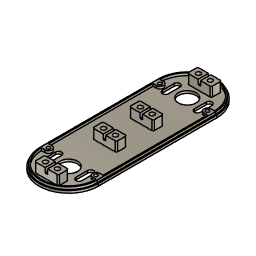
TRARM02_Link2A_100x50x2 (Autodesk Fusion 360 design; units mm, degrees)
Autodesk Fusion 360 part; units mm, degrees
sketch "스케치1" plane through (0, 0, 0) normal (0, 0, 1) x (1, 0, 0)
  line L0 (25, 100) -> (25, 0)
  line L1 (-25, 100) -> (-25, 0)
  arc A0 (25, 100) -> (-25, 100) centre (0, 100) ccw
  arc A1 (-25, 0) -> (25, 0) centre (0, 0) ccw
  dimension "d1" = 50
  dimension "d140" = 100
  constraint coincident A1.centre origin
  constraint vertical A1.centre A0.centre
  constraint vertical L0
  constraint tangent L1 A0
  constraint parallel L0 L1
  constraint horizontal A1.centre L1.end
  constraint horizontal A1.centre L0.end
  measures "d1" diameter of A1
  measures "d140" distance of L1.start L1.end
extrude "돌출1" add sketch "스케치1" along normal blind 2
sketch "스케치2" plane through (0, 0, 2) normal (0, 0, 1) x (-1, 0, 0)
  circle A0 centre (0, 0) radius 7.5
  circle A1 centre (0, -100) radius 7.5
  point P0 (25, -100)
  dimension "d150" = 100
  dimension "d151" = 15
  constraint coincident A0.centre origin
  constraint equal A0 A1
  constraint vertical A0.centre A1.centre
  measures "d150" distance of A0.centre A1.centre
  measures "d151" diameter of A0
extrude "돌출18" cut sketch "스케치2" against normal blind 2
sketch "스케치17" plane through (0, 0, 2) normal (0, 0, 1) x (-1, 0, 0)
  line L0 (10, -118.8) -> (-10, -118.8)
  line L1 (-10, -118.8) -> (-10, -110.2)
  line L2 (-10, -110.2) -> (10, -110.2)
  line L3 (10, -110.2) -> (10, -118.8)
  line L4 (10, -69.8) -> (-10, -69.8)
  line L5 (-10, -69.8) -> (-10, -61.2)
  line L6 (-10, -61.2) -> (10, -61.2)
  line L7 (10, -61.2) -> (10, -69.8)
  line L8 (10, -38.8) -> (-10, -38.8)
  line L9 (-10, -38.8) -> (-10, -30.2)
  line L10 (-10, -30.2) -> (10, -30.2)
  line L11 (10, -30.2) -> (10, -38.8)
  line L12 (10, 10.2) -> (-10, 10.2)
  line L13 (-10, 10.2) -> (-10, 18.8)
  line L14 (-10, 18.8) -> (10, 18.8)
  line L15 (10, 18.8) -> (10, 10.2)
  circle A0 centre (0, -100) radius 7.5
  circle A1 centre (-5, 14.5) radius 2.1 construction
  circle A2 centre (5, 14.5) radius 2.1 construction
  dimension "d154" = 20
  dimension "d160" = 10
  dimension "d161" = 10.2
  dimension "d162" = 10.2
  dimension "d163" = 30.2
  dimension "d164" = 30.2
  dimension "d165" = 4.2
  dimension "d166" = 14.5
  dimension "d167" = 10
  dimension "d168" = 5
  dimension "d169" = 4.3
  constraint horizontal L0
  constraint vertical L1
  constraint horizontal L2
  constraint vertical L3
  constraint horizontal L4
  constraint vertical L5
  constraint horizontal L6
  constraint vertical L7
  constraint horizontal L8
  constraint vertical L9
  constraint horizontal L10
  constraint vertical L11
  constraint horizontal L12
  constraint vertical L13
  constraint horizontal L14
  constraint vertical L15
  constraint equal L10 L14
  constraint equal L6 L10
  constraint equal L2 L6
  constraint equal L1 L5
  constraint equal L5 L9
  constraint vertical L6.end L10.end
  constraint vertical L10.end L14.end
  constraint vertical L2.end L6.end
  constraint equal L9 L13
  constraint equal A1 A2
  constraint horizontal A1.centre A2.centre
  measures "d154" distance of L13.end L14.end
  measures "d160" horizontal distance of origin L13.end
  measures "d161" vertical distance of origin L12.start
  measures "d162" vertical distance of L2.end A0.centre
  measures "d163" vertical distance of L4.start A0.centre
  measures "d164" vertical distance of origin L10.end
  measures "d165" diameter of A1
  measures "d166" vertical distance of origin A1.centre
  measures "d167" distance of A1.centre A2.centre
  measures "d168" horizontal distance of origin A1.centre
  measures "d169" vertical distance of L13.end A1.centre
extrude "돌출19" add sketch "스케치17" along normal blind 8 contours L0 L1 L2 L3 | L4 L5 L6 L7 | L8 L9 L10 L11 | L12 L13 L14 L15
sketch "스케치18" plane through (0, 0, 10) normal (0, 0, 1) x (-1, 0, 0)
  circle A0 centre (5, 14.5) radius 1.95
  circle A1 centre (-5, 14.5) radius 1.95
  circle A2 centre (-5, -34.5) radius 1.95
  circle A3 centre (5, -34.5) radius 1.95
  circle A4 centre (-5, -65.5) radius 1.95
  circle A5 centre (5, -65.5) radius 1.95
  circle A6 centre (5, -114.5) radius 1.95
  circle A7 centre (-5, -114.5) radius 1.95
  circle A8 centre (0, -100) radius 7.5
  line L0 (1, 10.2) -> (-1, 10.2)
  line L1 (-1, 10.2) -> (-1, 18.8)
  line L2 (-1, 18.8) -> (1, 18.8)
  line L3 (1, 18.8) -> (1, 10.2)
  line L4 (10, 10.2) -> (-10, 10.2)
  line L5 (-10, 18.8) -> (10, 18.8)
  line L6 (1, -30.2) -> (-1, -30.2)
  line L7 (-1, -30.2) -> (-1, -38.8)
  line L8 (-1, -38.8) -> (1, -38.8)
  line L9 (1, -38.8) -> (1, -30.2)
  line L10 (-10, -30.2) -> (10, -30.2)
  line L11 (10, -38.8) -> (-10, -38.8)
  line L12 (1, -69.8) -> (-1, -69.8)
  line L13 (-1, -69.8) -> (-1, -61.2)
  line L14 (-1, -61.2) -> (1, -61.2)
  line L15 (1, -61.2) -> (1, -69.8)
  line L16 (10, -69.8) -> (-10, -69.8)
  line L17 (-10, -61.2) -> (10, -61.2)
  line L18 (1, -118.8) -> (-1, -118.8)
  line L19 (-1, -118.8) -> (-1, -110.2)
  line L20 (-1, -110.2) -> (1, -110.2)
  line L21 (1, -110.2) -> (1, -118.8)
  line L22 (10, -118.8) -> (-10, -118.8)
  line L23 (-10, -110.2) -> (10, -110.2)
  dimension "d172" = 14.5
  dimension "d173" = 3.9
  dimension "d174" = 10
  dimension "d175" = 5
  dimension "d177" = 49
  dimension "d178" = 49
  dimension "d179" = 14.5
  dimension "d182" = 2
  dimension "d183" = 1
  constraint horizontal A0.centre A1.centre
  constraint equal A0 A1
  constraint vertical A4.centre A7.centre
  constraint vertical A2.centre A4.centre
  constraint vertical A1.centre A2.centre
  constraint equal A1 A4
  constraint equal A2 A4
  constraint equal A4 A7
  constraint equal A5 A6
  constraint equal A2 A3
  constraint vertical A5.centre A6.centre
  constraint vertical A3.centre A5.centre
  constraint vertical A0.centre A3.centre
  constraint horizontal A2.centre A3.centre
  constraint horizontal A4.centre A5.centre
  constraint horizontal A6.centre A7.centre
  constraint equal A6 A7
  constraint horizontal L0
  constraint vertical L1
  constraint horizontal L2
  constraint vertical L3
  constraint coincident L1.end L5
  constraint coincident L0.start L4
  constraint horizontal L6
  constraint vertical L7
  constraint horizontal L8
  constraint vertical L9
  constraint coincident L7.end L11
  constraint coincident L6.start L10
  constraint vertical L0.end L6.end
  constraint vertical L0.start L6.start
  constraint horizontal L12
  constraint vertical L13
  constraint horizontal L14
  constraint vertical L15
  constraint coincident L13.end L17
  constraint coincident L12.start L16
  constraint vertical L7.end L13.end
  constraint vertical L8.end L14.end
  constraint horizontal L18
  constraint vertical L19
  constraint horizontal L20
  constraint vertical L21
  constraint coincident L19.end L23
  constraint coincident L18.start L22
  constraint vertical L12.end L19.end
  constraint vertical L12.start L20.end
  measures "d172" vertical distance of origin A1.centre
  measures "d173" diameter of A1
  measures "d174" distance of A0.centre A1.centre
  measures "d175" horizontal distance of origin A1.centre
  measures "d177" distance of A0.centre A3.centre
  measures "d178" distance of A5.centre A6.centre
  measures "d179" vertical distance of A7.centre A8.centre
  measures "d182" distance of L1.end L2.end
  measures "d183" horizontal distance of origin L1.end
extrude "돌출20" cut sketch "스케치18" against normal blind 5 contours A0 | A1 | A2 | A3 | A4 | A5 | A6 | A7
extrude "돌출21" cut sketch "스케치18" against normal blind 4 contours L0 L1 L2 L3 L4 L5 | L6 L7 L8 L9 L10 L11 | L12 L13 L14 L15 L16 L17 | L18 L19 L20 L21 L22 L23
sketch "스케치19" plane through (0, 0, 2) normal (0, 0, 1) x (-1, 0, 0)
  line L0 (25, -100) -> (25, 0) construction
  arc A0 (-25, -100) -> (25, -100) centre (0, -100) ccw construction
  line L1 (-25, 0) -> (-25, -100) construction
  arc A1 (25, 0) -> (-25, 0) centre (0, 0) ccw construction
  line L2 (24, -100) -> (24, 0)
  arc A2 (24, 0) -> (-24, 0) centre (0, 0) ccw
  line L3 (-24, 0) -> (-24, -100)
  arc A3 (-24, -100) -> (24, -100) centre (0, -100) ccw
  arc A4 (23, 0) -> (-23, 0) centre (0, 0) ccw
  line L4 (-23, -6) -> (-23, -94)
  arc A5 (-23, -100) -> (23, -100) centre (0, -100) ccw
  line L5 (-20, -6) -> (-23, -6)
  line L6 (-20, 0) -> (-23, 0)
  arc A6 (-20, -6) -> (-20, 0) centre (-20, -3) ccw
  line L7 (20, -6) -> (23, -6)
  line L8 (20, 0) -> (23, 0)
  line L9 (23, -94) -> (23, -6)
  arc A7 (20, 0) -> (20, -6) centre (20, -3) ccw
  line L10 (-20, -100) -> (-23, -100)
  line L11 (-20, -94) -> (-23, -94)
  arc A8 (-20, -100) -> (-20.0042, -94) centre (-20, -97) ccw
  line L12 (20, -100) -> (23, -100)
  line L13 (20, -94) -> (23, -94)
  arc A9 (20.0029, -94) -> (20, -100) centre (20, -97) ccw
  dimension "d186" = -1
  dimension "d192" = 6
  dimension "d193" = 3
  dimension "d195" = 20
  dimension "d196" = 20
  dimension "d198" = 3
  constraint equal A8 A9
  constraint equal A7 A9
  constraint equal A6 A7
  constraint horizontal A7.centre A6.centre
  constraint horizontal A9.centre A8.centre
  constraint vertical A7.centre A9.centre
  constraint vertical A6.centre A8.centre
  constraint perpendicular L4 L5
  constraint perpendicular L4 L6
  constraint concentric A1 A4
  constraint concentric A0 A5
  constraint tangent A4 L9
  constraint tangent A4 L4
  constraint tangent L4 A5
  constraint tangent A5 L9
  constraint perpendicular L7 L9
  constraint perpendicular L8 L9
  constraint equal L7 L8
  constraint equal L6 L7
  constraint equal L5 L6
  constraint coincident L11.start A8
  constraint perpendicular L4 L11
  constraint coincident L11 A8.end
  constraint coincident L13.start A9
  constraint perpendicular L9 L13
  constraint coincident L13 A9.start
  constraint equal L10 L11
  constraint equal L5 L10
  constraint horizontal A5.start A0.centre
  constraint horizontal A0.centre A5.end
  constraint horizontal L10
  constraint horizontal L12
  constraint equal L12 L13
  measures "d192" diameter of A6
  measures "d193" vertical distance of A1.centre A6.centre
  measures "d195" horizontal distance of A1.centre A6.centre
  measures "d196" horizontal distance of A1.centre A7.centre
  measures "d198" distance of L5.start L4.start
extrude "돌출22" add sketch "스케치19" along normal blind 2
sketch "스케치21" plane through (0, 0, 4) normal (0, 0, 1) x (-1, 0, 0)
  circle A0 centre (-20, -3) radius 1.5
  circle A1 centre (20, -3) radius 1.5
  circle A2 centre (-20, -97) radius 1.5
  arc A3 (-20, -100) -> (-20.0042, -94) centre (-20, -97) ccw
  circle A4 centre (20, -97) radius 1.5
  arc A5 (20.0029, -94) -> (20, -100) centre (20, -97) ccw
  arc A6 (-20, -6) -> (-20, 0) centre (-20, -3) ccw
  arc A7 (20, 0) -> (20, -6) centre (20, -3) ccw
  dimension "d199" = 3
  constraint concentric A2 A3
  constraint concentric A4 A5
  constraint equal A2 A4
  constraint equal A0 A2
  constraint equal A0 A1
  constraint concentric A0 A6
  constraint concentric A1 A7
  measures "d199" diameter of A0
extrude "돌출24" cut sketch "스케치21" against normal blind 4
chamfer "챔퍼5" distance 2 angle 45 4 edges at (21.3985, 3.5424, 0) (-18.6015, 3.5424, 0) (-18.6015, 97.5424, 0) (21.3985, 97.5424, 0)
fillet "필렛4" radius 1 16 edges at (10, -18.8, 6) (10, -10.2, 6) (10, 30.2, 6) (10, 38.8, 6) (10, 61.2, 6) (10, 69.8, 6) (10, 110.2, 6) (10, 118.8, 6) (-10, 118.8, 6) (-10, 110.2, 6) (-10, 69.8, 6) (-10, 61.2, 6) (-10, 38.8, 6) (-10, 30.2, 6) (-10, -10.2, 6) (-10, -18.8, 6)
sketch "스케치23" plane through (0, 0, 2) normal (0, 0, 1) x (-1, 0, 0)
  line L0 (-16, -5) -> (-16, 5)
  line L1 (-11, -5) -> (-11, 5)
  arc A0 (-16, -5) -> (-11, -5) centre (-13.5, -5) ccw
  arc A1 (-11, 5) -> (-16, 5) centre (-13.5, 5) ccw
  arc A2 (16, 5) -> (11, 5) centre (13.5, 5) ccw
  line L2 (11, -5) -> (11, 5)
  line L3 (16, -5) -> (16, 5)
  arc A3 (11, -5) -> (16, -5) centre (13.5, -5) ccw
  arc A4 (-11, -95) -> (-16, -95) centre (-13.5, -95) ccw
  line L4 (-16, -105) -> (-16, -95)
  arc A5 (-16, -105) -> (-11, -105) centre (-13.5, -105) ccw
  line L5 (-11, -105) -> (-11, -95)
  arc A6 (16, -95) -> (11, -95) centre (13.5, -95) ccw
  line L6 (11, -105) -> (11, -95)
  line L7 (16, -105) -> (16, -95)
  arc A7 (11, -105) -> (16, -105) centre (13.5, -105) ccw
  dimension "d212" = 10
  dimension "d213" = 2.5
  dimension "d214" = 5
  dimension "d215" = 13.5
  dimension "d216" = 10
  dimension "d218" = 13.5
  dimension "d221" = 10
  dimension "d222" = 2.5
  dimension "d223" = 10
  dimension "d224" = 95
  constraint equal A0 A1
  constraint tangent L0 A0
  constraint tangent L1 A1
  constraint tangent L0 A1
  constraint tangent L1 A0
  constraint vertical A0.centre A1.centre
  constraint equal A2 A3
  constraint tangent L2 A3
  constraint tangent A2 L3
  constraint tangent A2 L2
  constraint tangent L3 A3
  constraint vertical A3.centre A2.centre
  constraint horizontal A1.centre A2.centre
  constraint equal A0 A3
  constraint equal A4 A5
  constraint tangent L4 A5
  constraint tangent A4 L5
  constraint tangent A4 L4
  constraint tangent A5 L5
  constraint vertical A5.centre A4.centre
  constraint equal A6 A7
  constraint tangent L6 A7
  constraint tangent A6 L7
  constraint tangent A6 L6
  constraint tangent L7 A7
  constraint vertical A7.centre A6.centre
  constraint horizontal A4.centre A6.centre
  constraint equal A5 A7
  constraint vertical A0.centre A4.centre
  constraint vertical A3.centre A6.centre
  measures "d212" vertical distance of A0.centre A1.centre
  measures "d213" radius of A0
  measures "d214" vertical distance of origin A0.centre
  measures "d215" horizontal distance of origin A0.centre
  measures "d216" vertical distance of A3.centre A2.centre
  measures "d218" horizontal distance of origin A2.centre
  measures "d221" vertical distance of A5.centre A4.centre
  measures "d222" radius of A5
  measures "d223" vertical distance of A7.centre A6.centre
  measures "d224" vertical distance of origin A4.centre
extrude "돌출26" cut sketch "스케치23" against normal blind 2
